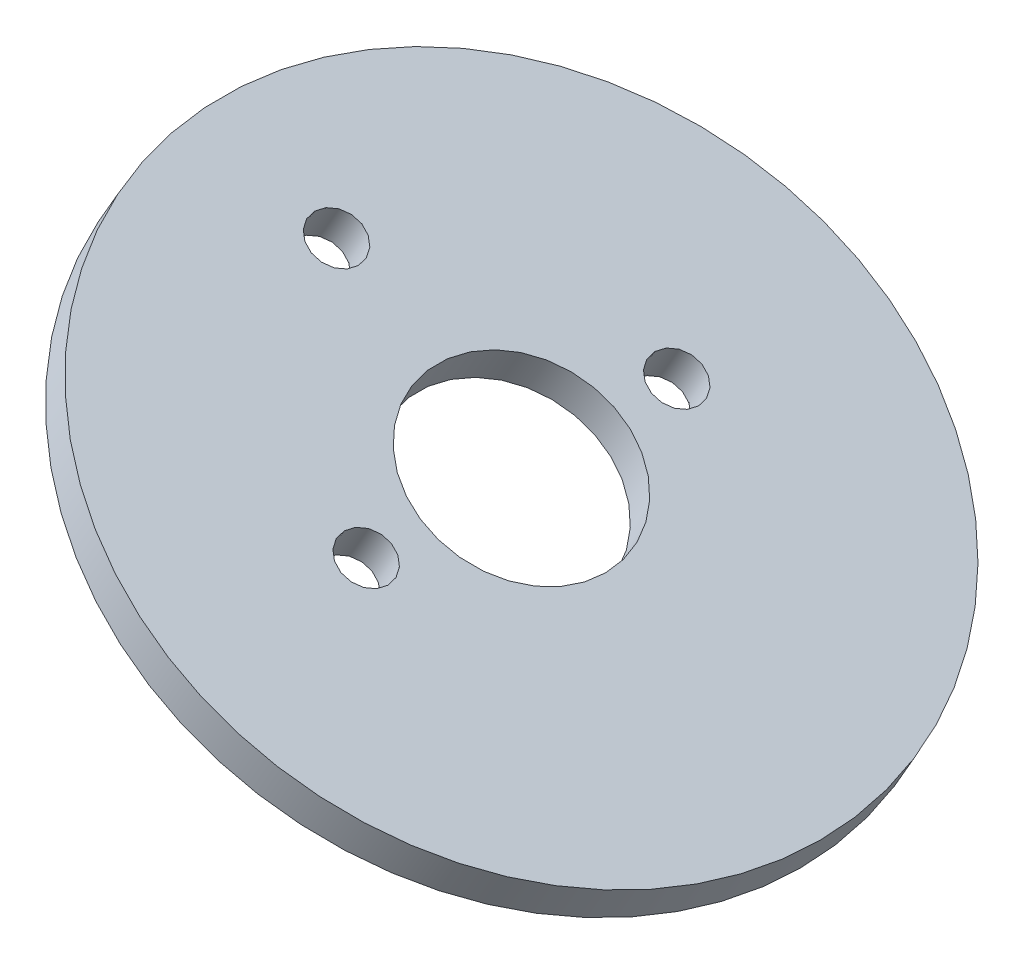
# Autodesk Inventor part: Head3MotorsSustain
Saved by Autodesk Inventor 2026 (Build 300175050, 175E)
## iProperties
Created: 2025-07-17
Part Number: Head3MotorsSustain
Material: Generic
Document SubType Name: Modeling
Designer: RubenPC
Density: 1 g/cm^3
Appearance: Default
Author: RubenPC
Autodesk Inventor part; units mm, degrees
ref_plane "YZ Plane" through (0, 0, 0) normal (1, 0, 0) x (0, 1, 0)
ref_plane "XZ Plane" through (0, 0, 0) normal (0, 1, 0) x (-1, 0, 0)
ref_plane "XY Plane" through (0, 0, 0) normal (0, 0, 1) x (1, 0, 0)
ref_plane "Work Plane1" through (47.25, -19.7742, 20) normal (-0.5, -0.8660254, 0) x (0.8660254, -0.5, 0)
sketch "Sketch1" plane through (47.25, -19.7742, 20) normal (-0.5, -0.8660254, 0) x (0.8660254, -0.5, 0)
  circle A0 centre (0, 0) radius 13.35 projected
  circle A1 centre (0, -8) radius 1.3 projected
  circle A2 centre (0, 8) radius 1.3 projected
  circle A3 centre (-11, 0) radius 1.3 projected
  circle A4 centre (0, 0) radius 5 projected
  circle A5 centre (0, 0) radius 17.78
  point P0 (-50.8068, -20)
  dimension "d0" = 35.56
  constraints: 1 centre point, 1 coincident
  measures "d0" diameter of A5
extrude "Extrusion1" add sketch "Sketch1" along normal blind 2 contours A0 | A5
body "Solid1"
